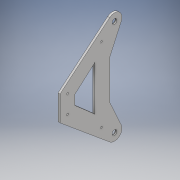
# Autodesk Inventor part: BaseCenterPlate
Saved by Autodesk Inventor 2018 (Build 220112000, 112)
## iProperties
Created: 2017-06-01
Part Number: BaseCenterPlate
Material: Generic
Document SubType Name: Modeling
Designer: Damian
Density: 1 g/cm^3
Appearance: Default
Author: Damian
Autodesk Inventor part; units mm, degrees
ref_plane "YZ Plane" through (0, 0, 0) normal (1, 0, 0) x (0, 1, 0)
ref_plane "XZ Plane" through (0, 0, 0) normal (0, 1, 0) x (-1, 0, 0)
ref_plane "XY Plane" through (0, 0, 0) normal (0, 0, 1) x (1, 0, 0)
sketch "Sketch1" plane through (0, 0, 0) normal (1, 0, 0) x (0, 1, 0)
  line L0 (79.4172, -148.1416) -> (-70.5828, -23.1416)
  line L1 (-70.5828, -23.1416) -> (-70.5828, 26.8584)
  line L2 (-70.5828, 26.8584) -> (79.4172, 151.8584)
  line L3 (79.4172, 151.8584) -> (29.4172, 41.8584)
  line L4 (29.4172, 41.8584) -> (29.4172, -38.1416)
  line L5 (29.4172, -38.1416) -> (79.4172, -148.1416)
  line L6 (-0.5828, -43.1416) -> (-0.5828, 46.8584)
  line L7 (-0.5828, 46.8584) -> (-40.5828, 11.8584)
  line L8 (-40.5828, 11.8584) -> (-40.5828, -8.1416)
  line L9 (-40.5828, -8.1416) -> (-0.5828, -43.1416)
  point P0 (0, 0)
  dimension "d0" = 0
  dimension "d2" = 50
  dimension "d6" = 150
  dimension "d7" = 300
  dimension "d9" = 80
  dimension "d104" = 50
  dimension "d105" = 15
  dimension "d106" = 20
  dimension "d107" = 40
  dimension "d108" = 30
  dimension "d109" = 90
  constraints: 20 end point, 3 equal length, 3 vertical, 1 parallel
  measures "d0" horizontal distance of L2.end L0.start
  measures "d2" distance of L0.end L1.end
  measures "d6" horizontal distance of L0.end L0.start
  measures "d7" distance of L0.start L2.end
  measures "d9" distance of L3.end L4.end
  measures "d104" horizontal distance of L3.end L2.end
  measures "d105" vertical distance of L1.end L7.end
  measures "d106" distance of L7.end L8.end
  measures "d107" horizontal distance of L7.end L6.end
  measures "d108" horizontal distance of L1.end L7.end
  measures "d109" distance of L6.start L6.end
extrude "Extrusion2" add sketch "Sketch1" along normal blind 4
fillet "Fillet2" radius 15 2 edges at (2, 79.4172, -148.1416) (2, 79.4172, 151.8584)
hole "Hole11" at (0, 38.6064, -94.607) direction (1, 0, 0) diameter 10 end through all
hole "Hole12" at (0, 38.6064, 98.3238) direction (1, 0, 0) diameter 10 end through all
hole "Hole13" at (0, 38.6064, -94.607) direction (1, 0, 0) diameter 11.6 depth 0.8 tip angle 118
hole "Hole14" at (0, 38.6064, 98.3238) direction (1, 0, 0) diameter 11.6 depth 0.8 tip angle 118
hole "Hole15" at (4, 12.0826, 76.2206) direction (-1, 0, 0) diameter 4 depth 8
hole "Hole16" at (4, 12.0826, -72.5039) direction (-1, 0, 0) diameter 4 depth 8
hole "Hole17" at (4, -55.5828, -16.116) direction (-1, 0, 0) diameter 4 depth 8
hole "Hole18" at (4, -55.5828, 19.8328) direction (-1, 0, 0) diameter 4 depth 8
body "Solid2"
